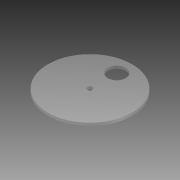
# Autodesk Inventor part: OpenROV 2_2 Dev EndCap 94
Saved by Autodesk Inventor 2015 (Build 190159000, 159)
## iProperties
Created: 2011-09-29
Part Number: OpenROV 2_2 Dev EndCap 94
Document SubType Name: Modeling
Designer: user
Density: 1 g/cm^3
Material: Generic
Appearance: Polycarbonate - Clear
Author: user
Autodesk Inventor part; units mm, degrees
ref_plane "YZ Plane" through (0, 0, 0) normal (1, 0, 0) x (0, 1, 0)
ref_plane "XZ Plane" through (0, 0, 0) normal (0, 1, 0) x (-1, 0, 0)
ref_plane "XY Plane" through (0, 0, 0) normal (0, 0, 1) x (1, 0, 0)
sketch "Sketch1" plane through (0, 0, 0) normal (0, 0, 1) x (1, 0, 0)
  circle A0 centre (0, 0) radius 49
  circle A1 centre (0, 0) radius 2.95
  circle A2 centre (0, 30) radius 10
  dimension "d0" = 98
  dimension "d1" = 5.9
  dimension "d4" = 20
  dimension "d5" = 30
  constraints: 3 centre point, 2 coincident
  measures "d0" diameter of A0
  measures "d1" diameter of A1
  measures "d4" diameter of A2
  measures "d5" distance of A1.centre A2.centre
extrude "Extrusion2" add sketch "Sketch1" along normal blind 3
body "Solid2"
